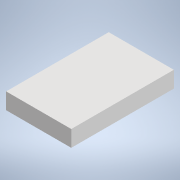
# Autodesk Inventor part: trussSeparator
Saved by Autodesk Inventor 2021 (Build 250183000, 183)
## iProperties
Created: 2021-06-06
Part Number: trussSeparator
Material: Generic
Document SubType Name: Modeling
Designer: Watchdog
Density: 1 g/cm^3
Appearance: Default
Mass: 64 g
Surface Area: 112 cm^2
Volume: 64 cm^3
Author: Watchdog
Autodesk Inventor part; units mm, degrees
ref_plane "YZ Plane" through (0, 0, 0) normal (1, 0, 0) x (0, 1, 0)
ref_plane "XZ Plane" through (0, 0, 0) normal (0, 1, 0) x (-1, 0, 0)
ref_plane "XY Plane" through (0, 0, 0) normal (0, 0, 1) x (1, 0, 0)
sketch "Sketch1" plane through (0, 0, 0) normal (0, 1, 0) x (-1, 0, 0)
  line L0 (20, 31.5) -> (-20, 31.5)
  line L1 (-20, 31.5) -> (-20, -31.5)
  line L2 (-20, -31.5) -> (20, -31.5)
  line L3 (20, -31.5) -> (20, 31.5)
  point P0 (0, 0)
  dimension "d0" = 63
  dimension "d1" = 31.5
  dimension "d2" = 40
  dimension "d3" = 20
  constraints: 8 end point, 2 parallel, 1 horizontal, 1 perpendicular
  measures "d0" distance between parallel lines of L2 L0
  measures "d1" distance from line of point (0, 0) L2
  measures "d2" distance between parallel lines of L1 L3
  measures "d3" distance from line of point (0, 0) L3
extrude "Extrusion1" add sketch "Sketch1" along normal blind 10
equation "\"d1\" = 0.5 * d0"
equation "\"d3\" = 0.5 * d2"
body "Solid1"
